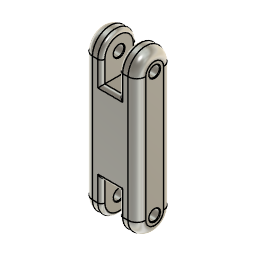
proximal v1 (Autodesk Fusion 360 design; units mm, degrees)
Autodesk Fusion 360 part; units mm, degrees
sketch "Çizim1" plane through (0, 0, 0) normal (0, 1, 0) x (1, 0, 0)
  line L0 (-15, 45) -> (15, 45)
  line L1 (15, 45) -> (15, -45)
  line L2 (15, -45) -> (-15, -45)
  line L3 (-15, -45) -> (-15, 45)
  line L4 (-15, 45) -> (15, -45) construction
  line L5 (15, 45) -> (-15, -45) construction
  dimension "d1" = 30
  dimension "d2" = 90
  constraint horizontal L0
  constraint perpendicular L0 L1
  constraint parallel L0 L2
  constraint parallel L1 L3
  constraint coincident L4 origin
  constraint coincident L5 origin
  measures "d1" distance of L1.end L2.end
  measures "d2" distance of L0.end L1.end
extrude "Ekstrüzyon1" add sketch "Çizim1" along normal blind 20
sketch "Çizim2" plane through (0, 0, 0) normal (0, -1, 0) x (1, 0, 0)
  line L0 (15, 45) -> (-15, 45)
  line L1 (-15, 45) -> (-15, -45)
  line L2 (-15, -45) -> (15, -45)
  line L3 (15, -45) -> (15, 45)
  line L4 (-5, 67) -> (5, 67)
  line L5 (5, 67) -> (5, 23)
  line L6 (5, 23) -> (-5, 23)
  line L7 (-5, 23) -> (-5, 67)
  line L8 (-5, 67) -> (5, 23) construction
  line L9 (5, 67) -> (-5, 23) construction
  point P0 (0, 45)
  dimension "d5" = 10
  dimension "d6" = 44
  constraint horizontal L4
  constraint perpendicular L4 L5
  constraint parallel L4 L6
  constraint parallel L5 L7
  constraint coincident L8 P0
  constraint coincident L9 P0
  constraint midpoint L0 P0
  measures "d5" distance of L5.end L6.end
  measures "d6" distance of L4.end L5.end
extrude "Ekstrüzyon2" cut sketch "Çizim2" against normal blind 70 contours L0 L5 L6 L7
sketch "Çizim3" plane through (0, 0, 0) normal (0, -1, 0) x (1, 0, 0)
  line L0 (-5, 23) -> (-5, 45)
  line L1 (-5, 45) -> (-15, 45)
  line L2 (-15, 45) -> (-15, -45)
  line L3 (-15, -45) -> (15, -45)
  line L4 (15, -45) -> (15, 45)
  line L5 (15, 45) -> (5, 45)
  line L6 (5, 45) -> (5, 23)
  line L7 (5, 23) -> (-5, 23)
  line L8 (-5, -23) -> (5, -23)
  line L9 (5, -23) -> (5, -67)
  line L10 (5, -67) -> (-5, -67)
  line L11 (-5, -67) -> (-5, -23)
  line L12 (-5, -23) -> (5, -67) construction
  line L13 (5, -23) -> (-5, -67) construction
  point P0 (0, -45)
  dimension "d9" = 10
  dimension "d10" = 44
  constraint horizontal L8
  constraint perpendicular L8 L9
  constraint parallel L8 L10
  constraint parallel L9 L11
  constraint coincident L12 P0
  constraint coincident L13 P0
  constraint midpoint L3 P0
  measures "d9" distance of L9.end L10.end
  measures "d10" distance of L8.end L9.end
extrude "Ekstrüzyon3" cut sketch "Çizim3" against normal blind 210 contours L3 L8 L9 L11
sketch "Çizim4" plane through (15, 0, 0) normal (1, 0, 0) x (0, 1, 0)
  line L0 (0, 45) -> (0, -45)
  line L1 (0, -45) -> (20, -45)
  line L2 (20, -45) -> (20, 45)
  line L3 (20, 45) -> (0, 45)
  circle A0 centre (10, 35) radius 10
  circle A1 centre (10, -35) radius 10
  circle A2 centre (10, 35) radius 3
  circle A3 centre (10, -35) radius 3
  dimension "d13" = 20
  dimension "d14" = 20
  dimension "d15" = 6
  dimension "d16" = 6
  constraint concentric A0 A2
  constraint concentric A1 A3
  measures "d13" diameter of A0
  measures "d14" diameter of A1
  measures "d15" diameter of A2
  measures "d16" diameter of A3
extrude "Ekstrüzyon4" cut sketch "Çizim4" against normal blind 52 contours A2 | A3
extrude "Ekstrüzyon5" cut sketch "Çizim4" against normal blind 115 contours L0 L3 A0 | L2 L3 A0 | L0 L1 A1 | L1 L2 A1
fillet "Radyus1" radius 2 16 edges at (-5, 20, 29) (-5, 10, 45) (-5, 0, 29) (5, 0, 29) (5, 10, 45) (5, 20, 29) (5, 0, -29) (5, 10, -45) (5, 20, -29) (-5, 20, -29) (-5, 10, -45) (-5, 0, -29) (0, 0, -23) (0, 0, 23) (0, 20, 23) (0, 20, -23)
fillet "Radyus2" radius 5 8 edges at (15, 10, 45) (15, 20, 0) (15, 10, -45) (15, 0, 0) (-15, 10, -45) (-15, 20, 0) (-15, 10, 45) (-15, 0, 0)
fillet "Radyus3" radius 0.3 8 edges at (-5, 7.203, 36.0848) (-15, 7.203, 33.9152) (5, 7.203, 33.9152) (15, 7.203, 36.0848) (15, 7.203, -33.9152) (5, 7.203, -36.0848) (-5, 7.203, -33.9152) (-15, 7.203, -36.0848)
